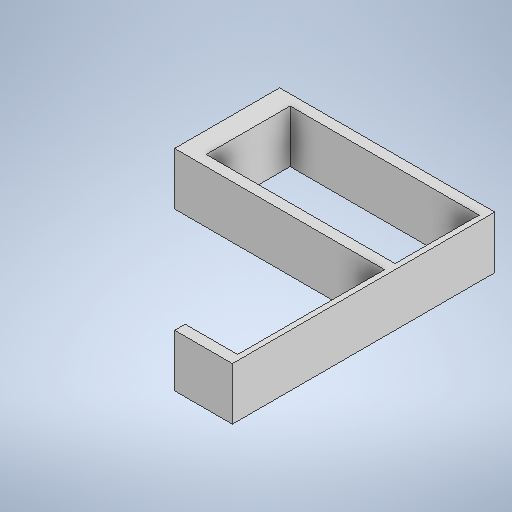
# Autodesk Inventor part: Part1
Saved by Autodesk Inventor 2025.2 (Build 292293000, 293)
## iProperties
Created: 2025-05-06
Part Number: Part1
Material: Generic
Document SubType Name: Sheet Metal
Designer: ziyuz
Density: 1 g/cm^3
Sheet Metal Rule: Default_mm
Appearance: Default
Author: ziyuz
Autodesk Inventor part; units mm, degrees
ref_plane "YZ Plane" through (0, 0, 0) normal (1, 0, 0) x (0, 1, 0)
ref_plane "XZ Plane" through (0, 0, 0) normal (0, 1, 0) x (-1, 0, 0)
ref_plane "XY Plane" through (0, 0, 0) normal (0, 0, 1) x (1, 0, 0)
sketch "Sketch1" plane through (0, 0, 0) normal (0, 1, 0) x (-1, 0, 0)
  line L0 (0, 0) -> (5, 0)
  line L1 (5, 0) -> (5, -250)
  line L2 (5, -250) -> (0, -250)
  line L3 (0, -250) -> (0, 0)
  line L4 (5, 0) -> (55, 0)
  line L5 (55, 0) -> (55, -10)
  line L6 (55, -10) -> (5, -10)
  line L7 (5, -10) -> (5, 0)
  line L8 (5, -10) -> (5, -160)
  line L9 (205, -160) -> (205, -170)
  line L10 (5, -170) -> (5, -160)
  line L11 (205, -250) -> (185, -250)
  line L12 (185, -250) -> (185, -150)
  line L13 (185, -150) -> (205, -150)
  line L14 (205, -150) -> (205, -250)
  line L15 (185, -150) -> (5, -150)
  line L16 (5, -150) -> (5, -160)
  line L17 (5, -160) -> (185, -160)
  line L18 (185, -250) -> (5, -250)
  line L19 (185, -250) -> (185, -240)
  line L20 (185, -240) -> (5, -240)
  point P0 (5, -150)
  dimension "d0" = 5
  dimension "d1" = 250
  dimension "d2" = 50
  dimension "d3" = 10
  dimension "d4" = 150
  dimension "d5" = 200
  dimension "d6" = 10
  dimension "d7" = 20
  dimension "d8" = 100
  dimension "d9" = 10
  dimension "d10" = 10
  constraints: 42 end point, 7 parallel, 6 perpendicular, 5 point on line, 3 horizontal, 1 collinear
  measures "d0" distance of L1.end L2.end
  measures "d1" distance of L0.end L1.end
  measures "d2" distance of L5.end L6.end
  measures "d3" distance of L4.end L5.end
  measures "d4" distance of L6.end L8.end
  measures "d5" distance of L9.end L10.start
  measures "d6" distance of L9.start L9.end
  measures "d7" distance of L12.end L13.end
  measures "d8" distance of L11.end L12.end
  measures "d9" distance of L15.end L8.end
  measures "d10" distance of L11.end L19.end
extrude "Extrusion1" add sketch "Sketch1" along normal blind 50 contours L0 L1 L2 L3 | L4 L5 L6 L1 | L1 L20 L12 L18 | L15 L12 L17 L1 | L12 L13 L14 L9 L11
equation "\"BendRadius\" = Thickness"
equation "\"BendReliefWidth\" = Thickness"
equation "\"BendReliefDepth\" = 0.5 * Thickness"
equation "\"CornerReliefSize\" = 4 * Thickness"
equation "\"MinimumRemnant\" = 2 * Thickness"
equation "\"TransitionRadius\" = BendRadius"
equation "\"JacobiRadiusSize\" = BendRadius"
equation "\"GapSize\" = Thickness"
equation "\"Thickness\" = 0.5"
body "Solid1"
